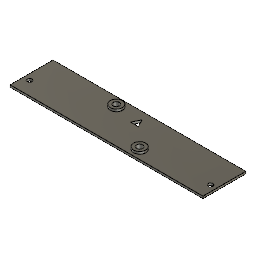
smmb_inner-bottom (Autodesk Fusion 360 design; units mm, degrees)
Autodesk Fusion 360 part; units mm, degrees
sketch "Sketch1" plane through (0, 0, 0) normal (0, 0, 1) x (1, 0, 0)
  line L0 (0, 0) -> (127.5, 0)
  line L1 (127.5, 0) -> (127.5, 28.5)
  line L2 (127.5, 28.5) -> (0, 28.5)
  line L3 (0, 28.5) -> (0, 0)
  circle A0 centre (4, 9) radius 1.55
  line L4 (63.75, 0) -> (63.75, 28.5) construction
  circle A1 centre (123.5, 9) radius 1.55
  line L5 (66.25, 18.5) -> (61.25, 18.5)
  line L6 (61.25, 18.5) -> (61.25, 23.5)
  line L7 (61.25, 23.5) -> (66.25, 23.5)
  line L8 (66.25, 23.5) -> (66.25, 18.5)
  line L9 (66.25, 18.5) -> (61.25, 23.5) construction
  line L10 (61.25, 18.5) -> (66.25, 23.5) construction
  line L11 (61.25, 18.5) -> (63.75, 23.5)
  line L12 (66.25, 18.5) -> (63.75, 23.5)
  point P0 (63.75, 21)
  dimension "d1" = 127.5
  dimension "d2" = 28.5
  dimension "d3" = 3.1
  dimension "d4" = 9
  dimension "d5" = 4
  dimension "d11" = 5
  dimension "d12" = 5
  dimension "d13" = 5
  constraint horizontal L0
  constraint vertical L1
  constraint horizontal L2
  constraint vertical L3
  constraint coincident L0.start L3.end
  constraint midpoint L0 L4.start
  constraint midpoint L2 L4.end
  constraint symmetric A0 L4 A1
  constraint perpendicular L5 L6
  constraint parallel L5 L7
  constraint parallel L6 L8
  constraint horizontal L5
  constraint coincident L9 P0
  constraint coincident L10 P0
  constraint coincident L4 P0
  constraint midpoint L7 L11.end
  measures "d1" distance of L0.start L0.end
  measures "d2" distance of L0.start L2.end
  measures "d3" diameter of A0
  measures "d4" distance of L0 A0.centre
  measures "d5" distance of L3 A0.centre
  measures "d11" distance of L5.end L6.end
  measures "d12" distance of L6.end L7.end
  measures "d13" distance of L2 L7
extrude "Extrude1" add sketch "Sketch1" along normal blind 1.5 contours L0 L1 L2 L3 | L7 L8 L12 | L6 L7 L11
sketch "Sketch2" plane through (0, 0, 1.5) normal (0, 0, 1) x (-1, 0, 0)
  circle A0 centre (-123.5, -9) radius 1.55
  circle A1 centre (-4, -9) radius 1.55
  line L0 (-66.25, -18.5) -> (-61.25, -18.5)
  line L1 (-61.25, -18.5) -> (-63.75, -23.5)
  line L2 (-63.75, -23.5) -> (-66.25, -18.5)
  line L3 (0, -28.5) -> (0, 0)
  line L4 (0, 0) -> (-127.5, 0)
  line L5 (-127.5, 0) -> (-127.5, -28.5)
  line L6 (-127.5, -28.5) -> (0, -28.5)
  line L7 (-63.75, -28.5) -> (-63.75, 0) construction
  line L8 (-87.75, -2.75) -> (-39.75, -2.75)
  line L9 (-39.75, -2.75) -> (-39.75, -25.75)
  line L10 (-39.75, -25.75) -> (-87.75, -25.75)
  line L11 (-87.75, -25.75) -> (-87.75, -2.75)
  line L12 (-87.75, -2.75) -> (-39.75, -25.75) construction
  line L13 (-39.75, -2.75) -> (-87.75, -25.75) construction
  circle A2 centre (-47.75, -22.55) radius 2.05
  circle A3 centre (-47.75, -22.55) radius 4.05
  circle A4 centre (-79.75, -5.95) radius 2.05
  circle A5 centre (-79.75, -5.95) radius 4.05
  point P0 (-63.75, -14.25)
  dimension "d14" = 48
  dimension "d15" = 23
  dimension "d18" = 8
  dimension "d19" = 3.2
  dimension "d20" = 4.1
  dimension "d21" = 8.1
  dimension "d22" = 4.1
  dimension "d23" = 8.1
  dimension "d24" = 8
  dimension "d25" = 3.2
  constraint midpoint L6 L7.start
  constraint midpoint L4 L7.end
  constraint perpendicular L8 L9
  constraint parallel L8 L10
  constraint parallel L9 L11
  constraint horizontal L8
  constraint coincident L12 P0
  constraint coincident L13 P0
  constraint midpoint L7 P0
  constraint concentric A2 A3
  constraint concentric A4 A5
  measures "d14" distance of L9.end L10.end
  measures "d15" distance of L8.end L9.end
  measures "d18" distance of L9 A2.centre
  measures "d19" distance of L10 A2.centre
  measures "d20" diameter of A2
  measures "d21" diameter of A3
  measures "d22" diameter of A4
  measures "d23" diameter of A5
  measures "d24" distance of L11 A4.centre
  measures "d25" distance of L8 A4.centre
extrude "Extrude2" add sketch "Sketch2" along normal blind 1.5 contours L8 A5 | L8 A5 | L10 A3 | L10 A3
extrude "Extrude3" cut sketch "Sketch2" against normal blind 1.5 contours A2 | A4
equation "d1 = 134 mm - 6 mm - 0.5 mm"
equation "d4 = 10.5 mm - 1.5 mm"
equation "d5 = 7 mm - 3 mm"
equation "d21 = d20 + 4 mm"
equation "d22 = d20"
equation "d23 = d21"
